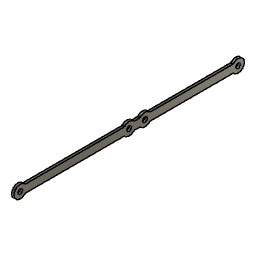
palito (Autodesk Fusion 360 design; units mm, degrees)
Autodesk Fusion 360 part; units mm, degrees
sketch "Boceto1" plane through (0, 0, 0) normal (1, 0, 0) x (0, 1, 0)
  line L0 (0, 0) -> (-0.8775, 0)
  line L1 (0, 5) -> (-0.8775, 5)
  line L2 (130, 0) -> (130.8775, 0)
  line L3 (130, 5) -> (130.8775, 5)
  arc A0 (-0.8775, 5) -> (-0.8775, 0) centre (-4, 2.5) ccw
  line L4 (78.1225, 0) -> (130, 0)
  line L5 (130, 5) -> (78.1225, 5)
  line L6 (75.0004, 5) -> (74.9996, 5)
  arc A1 (78.1225, 5) -> (71.8775, 5) centre (75, 2.5) ccw
  arc A2 (71.8775, 0) -> (78.1225, 0) centre (75, 2.5) ccw
  arc A3 (130.8775, 0) -> (130.8775, 5) centre (134, 2.5) ccw
  line L7 (0, 0) -> (61.8775, 0)
  line L8 (71.8775, 5) -> (68.1225, 5)
  line L9 (61.8775, 5) -> (0, 5)
  arc A4 (61.8775, 0) -> (68.1225, 0) centre (65, 2.5) ccw
  arc A5 (68.1225, 5) -> (61.8775, 5) centre (65, 2.5) ccw
  line L10 (0, 0) -> (65, 0)
  line L11 (68.1225, 0) -> (71.8775, 0)
  line L12 (0, 0) -> (61.8775, 0)
  line L13 (68.1225, 0) -> (71.8775, 0)
  circle A6 centre (-4, 2.5) radius 1.5
  circle A7 centre (65, 2.5) radius 1.5
  circle A8 centre (75, 2.5) radius 1.5
  circle A9 centre (134, 2.5) radius 1.5
  dimension "d1" = 130
  dimension "d2" = 5
  dimension "d7" = 8
  dimension "d9" = 65
  dimension "d10" = 2.5
  dimension "d11" = 8
  dimension "d15" = 3
  dimension "d16" = 3
  dimension "d17" = 3
  dimension "d18" = 3
  constraint horizontal L12
  constraint horizontal L5
  constraint coincident L0.start L7.start
  constraint coincident A2.start A1
  constraint collinear L4 L12
  constraint collinear L5 L6
  constraint collinear L6 L8
  constraint concentric A1 A2
  constraint coincident L9.start L8
  constraint coincident L7.end L10
  constraint collinear L8 L9
  constraint coincident L8.end A4
  constraint coincident A4.end L10
  constraint concentric A4 A5
  constraint collinear L10 L11
  constraint collinear L12 L13
  constraint concentric A0 A6
  constraint concentric A1 A8
  measures "d1" distance of L0.start L2.start
  measures "d2" distance of L0.start L1.start
  measures "d7" diameter of A1
  measures "d9" distance of L0.start L10.end
  measures "d10" distance of L10.end A4.centre
  measures "d11" diameter of A4
  measures "d15" diameter of A6
  measures "d16" diameter of A7
  measures "d17" diameter of A8
  measures "d18" diameter of A9
extrude "Extruir2" add sketch "Boceto1" along normal blind 1.5
